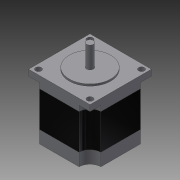
# Autodesk Inventor part: NEMA 23
Saved by Autodesk Inventor 2015 (Build 190159000, 159)
## iProperties
Created: 2017-01-20
Part Number: NEMA 23
Material: Generic
Document SubType Name: Modeling
Designer: Ernest
Density: 1 g/cm^3
Appearance: Default
Author: Ernest
Autodesk Inventor part; units mm, degrees
ref_plane "YZ Plane" through (0, 0, 0) normal (1, 0, 0) x (0, 1, 0)
ref_plane "XZ Plane" through (0, 0, 0) normal (0, 1, 0) x (-1, 0, 0)
ref_plane "XY Plane" through (0, 0, 0) normal (0, 0, 1) x (1, 0, 0)
sketch "Sketch1" plane through (0, 0, 0) normal (0, 0, 1) x (1, 0, 0)
  line L0 (18.25, -28.25) -> (-18.25, -28.25)
  line L1 (-28.25, -18.25) -> (-28.25, 18.25)
  line L2 (-18.25, 28.25) -> (18.25, 28.25)
  line L3 (28.25, 18.25) -> (28.25, -18.25)
  line L4 (28.25, -28.25) -> (-28.25, 28.25) construction
  line L5 (-28.25, -28.25) -> (28.25, 28.25) construction
  arc A0 (-28.25, 18.25) -> (-18.25, 28.25) centre (-28.25, 28.25) ccw
  arc A1 (18.25, 28.25) -> (28.25, 18.25) centre (28.25, 28.25) ccw
  arc A2 (-18.25, -28.25) -> (-28.25, -18.25) centre (-28.25, -28.25) ccw
  arc A3 (28.25, -18.25) -> (18.25, -28.25) centre (28.25, -28.25) ccw
  point P0 (0, 0)
  dimension "d0" = 56.5
  dimension "d1" = 56.5
  dimension "d2" = 20
  dimension "d3" = 20
  dimension "d4" = 20
  dimension "d5" = 20
  dimension "d6" = 56.5
  dimension "d7" = 56.5
  dimension "d8" = 56.5
  dimension "d9" = 56.5
  dimension "d10" = 28.25
  dimension "d11" = 28.25
  dimension "d12" = 28.25
  dimension "d13" = 28.25
  constraints: 12 end point, 8 point on circle, 4 centre point, 4 coincident, 2 midpoint, 2 parallel, 1 horizontal, 1 perpendicular
  measures "d0" distance of L4.end L5.end
  measures "d1" distance of L5.end L4.start
  measures "d2" diameter of A0
  measures "d3" diameter of A1
  measures "d4" diameter of A2
  measures "d5" diameter of A3
  measures "d6" distance of L4.end L5.start
  measures "d7" distance of L4.start L5.start
  measures "d8" distance between parallel lines of L2 L0
  measures "d9" distance between parallel lines of L1 L3
  measures "d10" distance from line of point (0, 0) L1
  measures "d11" distance from line of point (0, 0) L2
  measures "d12" horizontal distance of point (0, 0) L4.end
  measures "d13" horizontal distance of point (0, 0) L4.end
extrude "Extrusion1" add sketch "Sketch1" along normal blind 11.5
sketch "Sketch2" plane through (0, 0, 11.5) normal (0, 0, 1) x (1, 0, 0)
  line L0 (18.25, 28.25) -> (-18.25, 28.25) projected
  arc A0 (-28.25, 18.25) -> (-18.25, 28.25) centre (-28.25, 28.25) ccw projected
  line L1 (-28.25, 18.25) -> (-28.25, -18.25) projected
  arc A1 (-18.25, -28.25) -> (-28.25, -18.25) centre (-28.25, -28.25) ccw projected
  line L2 (-18.25, -28.25) -> (18.25, -28.25) projected
  arc A2 (28.25, -18.25) -> (18.25, -28.25) centre (28.25, -28.25) ccw projected
  line L3 (28.25, -18.25) -> (28.25, 18.25) projected
  arc A3 (18.25, 28.25) -> (28.25, 18.25) centre (28.25, 28.25) ccw projected
  point P0 (0, 0)
extrude "Extrusion2" add sketch "Sketch2" along normal blind 32.5 separate body
sketch "Sketch3" plane through (0, 0, 44) normal (0, 0, 1) x (1, 0, 0)
  line L0 (18.25, 28.25) -> (-18.25, 28.25) projected
  arc A0 (-28.25, 18.25) -> (-18.25, 28.25) centre (-28.25, 28.25) ccw projected
  line L1 (-28.25, 18.25) -> (-28.25, -18.25) projected
  arc A1 (-18.25, -28.25) -> (-28.25, -18.25) centre (-28.25, -28.25) ccw projected
  line L2 (-18.25, -28.25) -> (18.25, -28.25) projected
  arc A2 (28.25, -18.25) -> (18.25, -28.25) centre (28.25, -28.25) ccw projected
  line L3 (28.25, -18.25) -> (28.25, 18.25) projected
  arc A3 (18.25, 28.25) -> (28.25, 18.25) centre (28.25, 28.25) ccw projected
  point P0 (0, 0)
extrude "Extrusion3" add sketch "Sketch3" along normal blind 5 separate body
sketch "Sketch4" plane through (0, 0, 49) normal (0, 0, 1) x (1, 0, 0)
  line L0 (18.25, 28.25) -> (-18.25, 28.25) projected
  arc A0 (-28.25, 18.25) -> (-18.25, 28.25) centre (-28.25, 28.25) ccw projected
  line L1 (-28.25, 18.25) -> (-28.25, -18.25) projected
  arc A1 (-18.25, -28.25) -> (-28.25, -18.25) centre (-28.25, -28.25) ccw projected
  line L2 (-18.25, -28.25) -> (18.25, -28.25) projected
  arc A2 (28.25, -18.25) -> (18.25, -28.25) centre (28.25, -28.25) ccw projected
  line L3 (28.25, -18.25) -> (28.25, 18.25) projected
  arc A3 (18.25, 28.25) -> (28.25, 18.25) centre (28.25, 28.25) ccw projected
  line L4 (-28.25, 28.25) -> (28.25, 28.25)
  line L5 (28.25, 28.25) -> (28.25, -28.25)
  line L6 (28.25, -28.25) -> (-28.25, -28.25)
  line L7 (-28.25, -28.25) -> (-28.25, 28.25)
  circle A4 centre (-23.7, -23.7) radius 2.65
  circle A5 centre (23.7, -23.7) radius 2.65
  circle A6 centre (-23.7, 23.7) radius 2.65
  circle A7 centre (23.7, 23.7) radius 2.65
  point P0 (0, 0)
  dimension "d22" = 5.3
  dimension "d24" = 1.9
  dimension "d25" = 1.9
  dimension "d28" = 47.4
  dimension "d31" = 47.4
  constraints: 8 end point, 4 centre point, 2 horizontal, 2 parallel, 1 perpendicular, 1 vertical, 6 other
  measures "d22" diameter of A4
  measures "d24" distance edge to line of A4 L6
  measures "d25" distance edge to line of A4 L7
  measures "d28" distance of A4.centre A5.centre
  measures "d31" distance of A4.centre A6.centre
extrude "Extrusion4" add sketch "Sketch4" along normal blind 5.5 bodies 3
sketch "Sketch5" plane through (0, 0, 54.5) normal (0, 0, 1) x (1, 0, 0)
  circle A0 centre (0, 0) radius 19.05
  circle A1 centre (0, 0) radius 3.15
  dimension "d36" = 38.1
  dimension "d37" = 6.3
  constraints: 2 centre point, 2 coincident
  measures "d36" diameter of A0
  measures "d37" diameter of A1
extrude "Extrusion5" add sketch "Sketch5" along normal blind 1.7 bodies 3
extrude "Extrusion6" add sketch "Sketch5" along normal blind 21.4 contours A1 bodies 3
body "Solid1"
body "Solid2"
body "Solid3"
